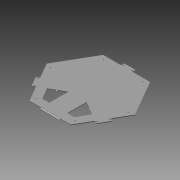
# Autodesk Inventor part: base_constr
Saved by Autodesk Inventor 2015 (Build 190159000, 159)
## iProperties
Created: 2015-04-17
Part Number: base_constr
Material: Ogólny
Document SubType Name: Modeling
Designer: Marcin
Density: 1 g/cm^3
Appearance: Domyślna
Author: Marcin
Autodesk Inventor part; units mm, degrees
ref_plane "YZ Plane" through (0, 0, 0) normal (1, 0, 0) x (0, 1, 0)
ref_plane "XZ Plane" through (0, 0, 0) normal (0, 1, 0) x (-1, 0, 0)
ref_plane "XY Plane" through (0, 0, 0) normal (0, 0, 1) x (1, 0, 0)
sketch "Szkic1" plane through (0, 0, 0) normal (0, 0, 1) x (1, 0, 0)
  line L0 (17.5, 0) -> (-17.5, 0)
  line L1 (-17.5, 0) -> (-17.5, 125)
  line L2 (-17.5, 125) -> (17.5, 125)
  line L3 (17.5, 125) -> (17.5, 0)
  line L4 (0, 0) -> (0, 163.4249) construction
  line L5 (-8.75, 15.1554) -> (8.75, -15.1554)
  line L6 (8.75, -15.1554) -> (-99.5032, -77.6554)
  line L7 (-99.5032, -77.6554) -> (-117.0032, -47.3446)
  line L8 (-117.0032, -47.3446) -> (-8.75, 15.1554)
  line L9 (0, 0) -> (-141.5301, -81.7124) construction
  line L10 (-8.75, -15.1554) -> (8.75, 15.1554)
  line L11 (8.75, 15.1554) -> (117.0032, -47.3446)
  line L12 (117.0032, -47.3446) -> (99.5032, -77.6554)
  line L13 (99.5032, -77.6554) -> (-8.75, -15.1554)
  line L14 (0, 0) -> (141.5301, -81.7124) construction
  dimension "d0" = 125
  dimension "d1" = 35
  dimension "d4" = 360
  constraints: 30 end point, 3 midpoint, 2 coincident, 2 parallel, 1 horizontal, 1 perpendicular, 1 vertical, 33 other
  measures "d0" distance of L2.end L0.start
  measures "d1" distance of L1.end L2.end
extrude "Wyciągnięcie proste1" add sketch "Szkic1" along normal blind 2
sketch "Szkic3" plane through (0, 0, 0) normal (0, 0, -1) x (-1, 0, 0)
  line L0 (-99.5032, -77.6554) -> (0, -20.2073) projected
  line L1 (0, -20.2073) -> (99.5032, -77.6554) projected
  line L2 (0, -20.2073) -> (0, -155.6549) construction
  line L3 (-90.9327, -72.7073) -> (-63.5085, -120.2073)
  line L4 (-63.5085, -120.2073) -> (0, -120.2073)
  line L5 (-49.0748, -95.2073) -> (0, -95.2073)
  line L6 (-49.0748, -95.2073) -> (-69.282, -60.2073)
  line L7 (90.9327, -72.7073) -> (63.5085, -120.2073)
  line L8 (63.5085, -120.2073) -> (0, -120.2073)
  line L9 (49.0748, -95.2073) -> (0, -95.2073)
  line L10 (49.0748, -95.2073) -> (69.282, -60.2073)
  line L11 (90.9327, -72.7073) -> (69.282, -60.2073)
  line L12 (-90.9327, -72.7073) -> (-69.282, -60.2073)
  point P0 (0, 0)
  dimension "d12" = 25
  dimension "d15" = 25
  dimension "d16" = 80
  dimension "d17" = 75
  constraints: 22 end point, 4 point on line, 4 symmetric about line, 2 perpendicular, 1 collinear, 1 horizontal, 1 parallel
  measures "d12" distance between parallel lines of L5 L4
  measures "d15" distance between parallel lines of L6 L3
  measures "d16" distance of L0.end L6.end
  measures "d17" distance of L0.end L5.end
extrude "Wyciągnięcie proste3" add sketch "Szkic3" against normal blind 2 contours L0 L6 L5 L9 L10 L1 L7 L8 L4 L3
sketch "Szkic5" plane through (0, 0, 2) normal (0, 0, 1) x (1, 0, 0)
  line L0 (-49.0748, -95.2073) -> (-69.282, -60.2073) projected
  line L1 (69.282, -60.2073) -> (49.0748, -95.2073) projected
  line L2 (-69.282, -60.2073) -> (0, -20.2073)
  line L3 (0, -20.2073) -> (69.282, -60.2073)
  line L4 (69.282, -60.2073) -> (49.0748, -95.2073)
  line L5 (-49.0748, -95.2073) -> (-69.282, -60.2073)
  line L6 (-90.9327, -72.7073) -> (-63.5085, -120.2073) projected
  line L7 (-63.5085, -120.2073) -> (63.5085, -120.2073) projected
  line L8 (63.5085, -120.2073) -> (90.9327, -72.7073) projected
  line L9 (-90.9327, -72.7073) -> (-63.5085, -120.2073)
  line L10 (63.5085, -120.2073) -> (-63.5085, -120.2073)
  line L11 (90.9327, -72.7073) -> (63.5085, -120.2073)
  line L12 (90.9327, -72.7073) -> (99.5032, -77.6554) projected
  line L13 (86.782, -29.8964) -> (17.5, 10.1036)
  line L14 (17.5, 10.1036) -> (17.5, 90.1036)
  line L15 (17.5, 90.1036) -> (57.9145, 90.1036)
  line L16 (106.9893, 5.1036) -> (86.782, -29.8964)
  line L17 (108.4327, -42.3964) -> (135.8568, 5.1036)
  line L18 (72.3483, 115.1036) -> (135.8568, 5.1036)
  line L19 (17.5, 115.1036) -> (72.3483, 115.1036)
  line L20 (-17.5, 90.1036) -> (-17.5, 10.1036)
  line L21 (-17.5, 10.1036) -> (-86.782, -29.8964)
  line L22 (-86.782, -29.8964) -> (-106.9893, 5.1036)
  line L23 (-57.9145, 90.1036) -> (-17.5, 90.1036)
  line L24 (-17.5, 115.1036) -> (-72.3483, 115.1036)
  line L25 (-135.8568, 5.1036) -> (-72.3483, 115.1036)
  line L26 (-108.4327, -42.3964) -> (-135.8568, 5.1036)
  line L27 (-106.9893, 5.1036) -> (-57.9145, 90.1036)
  line L28 (106.9893, 5.1036) -> (57.9145, 90.1036)
  line L29 (-108.4327, -42.3964) -> (-86.782, -29.8964)
  line L30 (-117.0032, -47.3446) -> (-17.5, 10.1036) projected
  line L31 (108.4327, -42.3964) -> (86.782, -29.8964)
  line L32 (17.5, 10.1036) -> (117.0032, -47.3446) projected
  line L33 (17.5, 90.1036) -> (17.5, 115.1036)
  line L34 (17.5, 125) -> (17.5, 10.1036) projected
  line L35 (-17.5, 90.1036) -> (-17.5, 115.1036)
  line L36 (-17.5, 10.1036) -> (-17.5, 125) projected
  point P0 (0, 0)
  dimension "d24" = 360
  constraints: 54 end point, 6 collinear, 1 horizontal, 1 perpendicular, 49 other
extrude "Wyciągnięcie proste5" add sketch "Szkic5" against normal blind 2 contours L16 L28 L15 L33 L19 L18 L17 L31 | L23 L27 L22 L29 L26 L25 L24 L35
sketch "Szkic6" plane through (0, 0, 2) normal (0, 0, 1) x (1, 0, 0)
  line L0 (-63.5085, -120.2073) -> (63.5085, -120.2073) projected
  line L1 (17.5, 10.1036) -> (17.5, 90.1036) projected
  line L2 (-17.5, 90.1036) -> (-17.5, 10.1036) projected
  line L3 (17.5, 10.1036) -> (-17.5, 10.1036)
  line L4 (-17.5, 10.1036) -> (-17.5, -120.2073)
  line L5 (-17.5, -120.2073) -> (17.5, -120.2073)
  line L6 (17.5, -120.2073) -> (17.5, 10.1036)
  point P0 (0, 0)
  constraints: 8 end point, 2 parallel, 1 collinear, 1 horizontal, 1 perpendicular, 1 point on line
extrude "Wyciągnięcie proste6" add sketch "Szkic6" against normal blind 2
sketch "Szkic7" plane through (0, 0, 0) normal (0, 0, -1) x (-1, 0, 0)
  line L0 (0, 0) -> (60, 103.923) construction
  line L1 (0, 0) -> (0, 71.3252)
  point P0 (-60, 103.923)
  point P1 (-120, 0)
  point P2 (-60, -103.923)
  point P3 (60, -103.923)
  point P4 (120, 0)
  dimension "d30" = 120
  dimension "d33" = 360
  dimension "d42" = 30
  constraints: 4 end point, 1 coincident, 1 vertical, 7 other
  measures "d30" distance of L0.start L0.end
  measures "d42" angle of L0 L1
hole "Otwór1" at (-60, 103.923, 0) at (60, 103.923, 0) at (120, 0, 0) at (60, -103.923, 0) at (-60, -103.923, 0) at (-120, 0, 0) direction (0, 0, 1) diameter 3 depth 8 tip angle 118
sketch "Szkic8" plane through (0, 0, 0) normal (0, 0, -1) x (-1, 0, 0)
  point P0 (-96.057, -71.6244)
  point P1 (-110.057, -47.3756)
  point P2 (-14, 119)
  point P3 (14, 119)
  point P4 (110.057, -47.3756)
  point P5 (96.057, -71.6244)
hole "Otwór2" at (96.057, -71.6244, 0) at (110.057, -47.3756, 0) at (14, 119, 0) at (-14, 119, 0) at (-110.057, -47.3756, 0) at (-96.057, -71.6244, 0) direction (0, 0, 1) diameter 3.4 depth 2
sketch "Szkic9" plane through (0, 0, 0) normal (0, 0, -1) x (-1, 0, 0)
  circle A0 centre (110.057, -47.3756) radius 1.7 projected
  circle A1 centre (-14, 119) radius 1.7 projected
  circle A2 centre (-96.057, -71.6244) radius 1.7 projected
  circle A3 centre (-110.057, -47.3756) radius 1.7 projected
  circle A4 centre (14, 119) radius 1.7 projected
  circle A5 centre (96.057, -71.6244) radius 1.7 projected
  circle A6 centre (60, -103.923) radius 1.5 projected
  circle A7 centre (-120, 0) radius 1.5 projected
  circle A8 centre (60, 103.923) radius 1.5 projected
  circle A9 centre (-60, 103.923) radius 1.5 projected
  circle A10 centre (-60, -103.923) radius 1.5 projected
  circle A11 centre (120, 0) radius 1.5 projected
  line L0 (-17.5, -95.2073) -> (-49.0748, -95.2073) projected
  line L1 (-49.0748, -95.2073) -> (-69.282, -60.2073) projected
  line L2 (-69.282, -60.2073) -> (-17.5, -30.3109) projected
  line L3 (-17.5, -30.3109) -> (-17.5, -95.2073) projected
  line L4 (-63.5085, -120.2073) -> (63.5085, -120.2073) projected
  line L5 (63.5085, -120.2073) -> (90.9327, -72.7073) projected
  line L6 (90.9327, -72.7073) -> (99.5032, -77.6554) projected
  line L7 (99.5032, -77.6554) -> (117.0032, -47.3446) projected
  line L8 (117.0032, -47.3446) -> (108.4327, -42.3964) projected
  line L9 (108.4327, -42.3964) -> (135.8568, 5.1036) projected
  line L10 (135.8568, 5.1036) -> (72.3483, 115.1036) projected
  line L11 (72.3483, 115.1036) -> (17.5, 115.1036) projected
  line L12 (17.5, 115.1036) -> (17.5, 125) projected
  line L13 (17.5, 125) -> (-17.5, 125) projected
  line L14 (-17.5, 125) -> (-17.5, 115.1036) projected
  line L15 (-17.5, 115.1036) -> (-72.3483, 115.1036) projected
  line L16 (-72.3483, 115.1036) -> (-135.8568, 5.1036) projected
  line L17 (-135.8568, 5.1036) -> (-108.4327, -42.3964) projected
  line L18 (-108.4327, -42.3964) -> (-117.0032, -47.3446) projected
  line L19 (-117.0032, -47.3446) -> (-99.5032, -77.6554) projected
  line L20 (-99.5032, -77.6554) -> (-90.9327, -72.7073) projected
  line L21 (-90.9327, -72.7073) -> (-63.5085, -120.2073) projected
  line L22 (17.5, -95.2073) -> (17.5, -30.3109) projected
  line L23 (17.5, -30.3109) -> (69.282, -60.2073) projected
  line L24 (69.282, -60.2073) -> (49.0748, -95.2073) projected
  line L25 (49.0748, -95.2073) -> (17.5, -95.2073) projected
  line L26 (17.5, 10.1036) -> (17.5, 90.1036) projected
  line L27 (17.5, 90.1036) -> (57.9145, 90.1036) projected
  line L28 (57.9145, 90.1036) -> (106.9893, 5.1036) projected
  line L29 (106.9893, 5.1036) -> (86.782, -29.8964) projected
  line L30 (86.782, -29.8964) -> (17.5, 10.1036) projected
  line L31 (-17.5, 10.1036) -> (-86.782, -29.8964) projected
  line L32 (-86.782, -29.8964) -> (-106.9893, 5.1036) projected
  line L33 (-106.9893, 5.1036) -> (-57.9145, 90.1036) projected
  line L34 (-57.9145, 90.1036) -> (-17.5, 90.1036) projected
  line L35 (-17.5, 90.1036) -> (-17.5, 10.1036) projected
  line L36 (-106.9893, 5.1036) -> (-57.9145, 90.1036) projected
  point P0 (0, 0)
extrude "Wyciągnięcie proste7" add sketch "Szkic9" against normal blind 2 contours L26 L27 L28 L29 L30 | L31 L32 L33 L34 L35
sketch "Szkic10" plane through (0, 0, 0) normal (0, 0, -1) x (-1, 0, 0)
  line L0 (-88.0852, 23.4319) -> (-70.7647, 13.4319) projected
  line L1 (-88.0852, 23.4319) -> (-89.0852, 21.6998) projected
  line L2 (-71.7647, 11.6998) -> (-89.0852, 21.6998) projected
  line L3 (-70.7647, 13.4319) -> (-71.7647, 11.6998) projected
  line L4 (-95.0852, 11.3075) -> (-57.3352, 76.6925) projected
  line L5 (-57.3352, 76.6925) -> (-59.0673, 77.6925) projected
  line L6 (-96.8173, 12.3075) -> (-59.0673, 77.6925) projected
  line L7 (-95.0852, 11.3075) -> (-96.8173, 12.3075) projected
  line L8 (-63.3352, 66.3002) -> (-46.0147, 56.3002) projected
  line L9 (-63.3352, 66.3002) -> (-64.3352, 64.5681) projected
  line L10 (-47.0147, 54.5681) -> (-64.3352, 64.5681) projected
  line L11 (-46.0147, 56.3002) -> (-47.0147, 54.5681) projected
  line L12 (-17.5, 104) -> (-37.5, 104) projected
  line L13 (-17.5, 104) -> (-17.5, 106) projected
  line L14 (-37.5, 106) -> (-17.5, 106) projected
  line L15 (-37.5, 104) -> (-37.5, 106) projected
  line L16 (-39.5, 113) -> (-39.5, 23) projected
  line L17 (-39.5, 23) -> (-37.5, 23) projected
  line L18 (-37.5, 113) -> (-37.5, 23) projected
  line L19 (-39.5, 113) -> (-37.5, 113) projected
  line L20 (-17.5, 30) -> (-37.5, 30) projected
  line L21 (-17.5, 30) -> (-17.5, 32) projected
  line L22 (-37.5, 32) -> (-17.5, 32) projected
  line L23 (-37.5, 30) -> (-37.5, 32) projected
  line L24 (-36.4628, -0.8446) -> (-46.4628, 16.476) projected
  line L25 (-36.4628, -0.8446) -> (-34.7308, 0.1554) projected
  line L26 (-44.7308, 17.476) -> (-34.7308, 0.1554) projected
  line L27 (-46.4628, 16.476) -> (-44.7308, 17.476) projected
  line L28 (-39.6686, 22.708) -> (-117.6109, -22.292) projected
  line L29 (-117.6109, -22.292) -> (-116.6109, -24.024) projected
  line L30 (-38.6686, 20.976) -> (-116.6109, -24.024) projected
  line L31 (-39.6686, 22.708) -> (-38.6686, 20.976) projected
  line L32 (-100.5487, -37.8446) -> (-110.5487, -20.524) projected
  line L33 (-100.5487, -37.8446) -> (-98.8166, -36.8446) projected
  line L34 (-108.8166, -19.524) -> (-98.8166, -36.8446) projected
  line L35 (-110.5487, -20.524) -> (-108.8166, -19.524) projected
  line L36 (14.6442, 35.013) -> (31.9647, 45.013) projected
  line L37 (14.6442, 35.013) -> (15.6442, 33.2809) projected
  line L38 (32.9647, 43.2809) -> (15.6442, 33.2809) projected
  line L39 (31.9647, 45.013) -> (32.9647, 43.2809) projected
  line L40 (36.6442, -3.0922) -> (53.9647, 6.9078) projected
  line L41 (36.6442, -3.0922) -> (37.6442, -4.8242) projected
  line L42 (54.9647, 5.1758) -> (37.6442, -4.8242) projected
  line L43 (53.9647, 6.9078) -> (54.9647, 5.1758) projected
  line L44 (64.9647, -12.1447) -> (21.9647, 62.3335) projected
  line L45 (23.6968, 63.3335) -> (66.6968, -11.1447) projected
  line L46 (23.6968, 63.3335) -> (21.9647, 62.3335) projected
  line L47 (66.6968, -11.1447) -> (64.9647, -12.1447) projected
  circle A0 centre (114.5602, 19.9534) radius 1.75 projected
  circle A1 centre (74.5602, 89.2354) radius 1.75 projected
  line L48 (52.2647, -45.4748) -> (51.2647, -47.2069) projected
  line L49 (52.2647, -45.4748) -> (34.9442, -35.4748) projected
  line L50 (34.9442, -35.4748) -> (33.9442, -37.2069) projected
  line L51 (33.9442, -37.2069) -> (51.2647, -47.2069) projected
  line L52 (67.5147, -19.0611) -> (69.2468, -20.0611) projected
  line L53 (69.2468, -20.0611) -> (51.9968, -49.9389) projected
  line L54 (51.9968, -49.9389) -> (50.2647, -48.9389) projected
  line L55 (50.2647, -48.9389) -> (51.2647, -47.2069) projected
  line L56 (51.2647, -47.2069) -> (33.9442, -37.2069) projected
  line L57 (34.9442, -35.4748) -> (33.9442, -37.2069) projected
  line L58 (34.9442, -35.4748) -> (52.2647, -45.4748) projected
  line L59 (52.2647, -45.4748) -> (65.5147, -22.5252) projected
  line L60 (48.1942, -12.5252) -> (65.5147, -22.5252) projected
  line L61 (48.1942, -12.5252) -> (49.1942, -10.7931) projected
  line L62 (66.5147, -20.7931) -> (49.1942, -10.7931) projected
  line L63 (66.5147, -20.7931) -> (67.5147, -19.0611) projected
  line L64 (-50.2647, -48.9389) -> (-51.9968, -49.9389) projected
  line L65 (-51.9968, -49.9389) -> (-69.2468, -20.0611) projected
  line L66 (-69.2468, -20.0611) -> (-67.5147, -19.0611) projected
  line L67 (-67.5147, -19.0611) -> (-66.5147, -20.7931) projected
  line L68 (-66.5147, -20.7931) -> (-49.1942, -10.7931) projected
  line L69 (-48.1942, -12.5252) -> (-49.1942, -10.7931) projected
  line L70 (-48.1942, -12.5252) -> (-65.5147, -22.5252) projected
  line L71 (-65.5147, -22.5252) -> (-52.2647, -45.4748) projected
  line L72 (-34.9442, -35.4748) -> (-52.2647, -45.4748) projected
  line L73 (-34.9442, -35.4748) -> (-33.9442, -37.2069) projected
  line L74 (-51.2647, -47.2069) -> (-33.9442, -37.2069) projected
  line L75 (-51.2647, -47.2069) -> (-50.2647, -48.9389) projected
  line L76 (1, -87.4073) -> (1, -62.4073) projected
  line L77 (-17.5, -60.4073) -> (17.5, -60.4073) projected
  line L78 (1, -62.4073) -> (17.5, -62.4073) projected
  line L79 (-1, -87.4073) -> (1, -87.4073) projected
  line L80 (-1, -62.4073) -> (-1, -87.4073) projected
  line L81 (-17.5, -62.4073) -> (-1, -62.4073) projected
  line L82 (28.5, -120.2073) -> (-28.5, -120.2073) projected
  line L83 (-28.5, -120.2073) -> (-28.5, -118.2073) projected
  line L84 (-18.5, -118.2073) -> (-28.5, -118.2073) projected
  line L85 (-18.5, -118.2073) -> (-18.5, -93.2073) projected
  line L86 (-18.5, -93.2073) -> (-16.5, -93.2073) projected
  line L87 (-16.5, -118.2073) -> (-16.5, -93.2073) projected
  line L88 (16.5, -118.2073) -> (-16.5, -118.2073) projected
  line L89 (16.5, -118.2073) -> (16.5, -93.2073) projected
  line L90 (18.5, -93.2073) -> (16.5, -93.2073) projected
  line L91 (18.5, -118.2073) -> (18.5, -93.2073) projected
  line L92 (28.5, -118.2073) -> (18.5, -118.2073) projected
  line L93 (28.5, -120.2073) -> (28.5, -118.2073) projected
  line L94 (-17.5, -62.4073) -> (-17.5, -60.4073)
  line L95 (-17.5, -95.2073) -> (-17.5, -30.3109) projected
  line L96 (17.5, -62.4073) -> (17.5, -60.4073)
  line L97 (17.5, -95.2073) -> (17.5, -30.3109) projected
  line L98 (-17.25, 68) -> (-17.25, 70) projected
  line L99 (-17.25, 70) -> (17.25, 70) projected
  line L100 (17.25, 70) -> (17.25, 68) projected
  line L101 (17.25, 68) -> (15.25, 68) projected
  line L102 (15.25, 68) -> (15.25, 48) projected
  line L103 (13.25, 48) -> (15.25, 48) projected
  line L104 (13.25, 48) -> (13.25, 68) projected
  line L105 (13.25, 68) -> (-13.25, 68) projected
  line L106 (-13.25, 48) -> (-13.25, 68) projected
  line L107 (-13.25, 48) -> (-15.25, 48) projected
  line L108 (-15.25, 68) -> (-15.25, 48) projected
  line L109 (-15.25, 68) -> (-17.25, 68) projected
  point P0 (0, 0)
  constraints: 4 end point, 2 collinear
sketch "Szkic11" plane through (0, 0, 0) normal (0, 0, -1) x (-1, 0, 0)
  circle A0 centre (110.057, -47.3756) radius 1.7 projected
  circle A1 centre (-14, 119) radius 1.7 projected
  circle A2 centre (-96.057, -71.6244) radius 1.7 projected
  circle A3 centre (-110.057, -47.3756) radius 1.7 projected
  circle A4 centre (14, 119) radius 1.7 projected
  circle A5 centre (96.057, -71.6244) radius 1.7 projected
  circle A6 centre (60, -103.923) radius 1.5 projected
  circle A7 centre (-120, 0) radius 1.5 projected
  circle A8 centre (60, 103.923) radius 1.5 projected
  circle A9 centre (-60, 103.923) radius 1.5 projected
  circle A10 centre (-60, -103.923) radius 1.5 projected
  circle A11 centre (120, 0) radius 1.5 projected
  line L0 (-17.5, -95.2073) -> (-49.0748, -95.2073) projected
  line L1 (-49.0748, -95.2073) -> (-69.282, -60.2073) projected
  line L2 (-69.282, -60.2073) -> (-17.5, -30.3109) projected
  line L3 (-17.5, -30.3109) -> (-17.5, -95.2073) projected
  line L4 (-63.5085, -120.2073) -> (63.5085, -120.2073) projected
  line L5 (63.5085, -120.2073) -> (90.9327, -72.7073) projected
  line L6 (90.9327, -72.7073) -> (99.5032, -77.6554) projected
  line L7 (99.5032, -77.6554) -> (117.0032, -47.3446) projected
  line L8 (117.0032, -47.3446) -> (108.4327, -42.3964) projected
  line L9 (108.4327, -42.3964) -> (135.8568, 5.1036) projected
  line L10 (135.8568, 5.1036) -> (72.3483, 115.1036) projected
  line L11 (72.3483, 115.1036) -> (17.5, 115.1036) projected
  line L12 (17.5, 115.1036) -> (17.5, 125) projected
  line L13 (17.5, 125) -> (-17.5, 125) projected
  line L14 (-17.5, 125) -> (-17.5, 115.1036) projected
  line L15 (-17.5, 115.1036) -> (-72.3483, 115.1036) projected
  line L16 (-72.3483, 115.1036) -> (-135.8568, 5.1036) projected
  line L17 (-135.8568, 5.1036) -> (-108.4327, -42.3964) projected
  line L18 (-108.4327, -42.3964) -> (-117.0032, -47.3446) projected
  line L19 (-117.0032, -47.3446) -> (-99.5032, -77.6554) projected
  line L20 (-99.5032, -77.6554) -> (-90.9327, -72.7073) projected
  line L21 (-90.9327, -72.7073) -> (-63.5085, -120.2073) projected
  line L22 (17.5, -95.2073) -> (17.5, -30.3109) projected
  line L23 (17.5, -30.3109) -> (69.282, -60.2073) projected
  line L24 (69.282, -60.2073) -> (49.0748, -95.2073) projected
  line L25 (49.0748, -95.2073) -> (17.5, -95.2073) projected
  line L26 (-17.5, -95.2073) -> (-27.5, -95.2073)
  line L27 (-49.0748, -95.2073) -> (-17.5, -95.2073) projected
  line L28 (-27.5, -95.2073) -> (-27.5, -36.0844)
  line L29 (-27.5, -36.0844) -> (-17.5, -30.3109)
  line L30 (-17.5, -30.3109) -> (-69.282, -60.2073) projected
  line L31 (-17.5, -30.3109) -> (-17.5, -95.2073)
  line L32 (17.5, -95.2073) -> (27.5, -95.2073)
  line L33 (17.5, -95.2073) -> (49.0748, -95.2073) projected
  line L34 (27.5, -95.2073) -> (27.5, -36.0844)
  line L35 (69.282, -60.2073) -> (17.5, -30.3109) projected
  line L36 (17.5, -30.3109) -> (27.5, -36.0844)
  line L37 (17.5, -30.3109) -> (17.5, -95.2073)
  point P0 (0, 0)
  dimension "d52" = 10
  dimension "d53" = 10
  constraints: 16 end point, 3 collinear, 3 point on line, 2 perpendicular, 1 parallel
  measures "d52" distance of L0.start L26.end
  measures "d53" distance of L22.start L32.end
extrude "Wyciągnięcie proste8" add sketch "Szkic11" against normal blind 2 contours L0 L28 L2 L3 | L22 L23 L34 L25
extrude "Wyciągnięcie proste9" cut sketch "Szkic10" against normal blind 2 contours L0 L3 L2 L1 | L1 L4 L7 L6 L5 | L4 L8 L11 L10 | L12 L15 L14 L13 | L18 L17 L16 L19 L15 | L22 L21 L20 L18 | L24 L27 L26 L25 | L30 L29 L28 L31 L27 | L34 L33 L32 L30 | L36 L39 L38 L37 | L44 L46 L45 L47 L43 L39 | L43 L42 L41 L40 | A0 | A1 | L59 L60 L61 L62 L63 L52 L53 L54 L55 L48 | L48 L51 L50 L49 | L64 L65 L66 L67 L68 L69 L70 L71 L72 L73 L74 L75 | L79 L80 L81 L94 L77 L96 L78 L76 | L90 L91 L92 L93 L82 L83 L84 L85 L86 L87 L88 L89 | L98 L99 L100 L101 L102 L103 L104 L105 L106 L107 L108 L109
